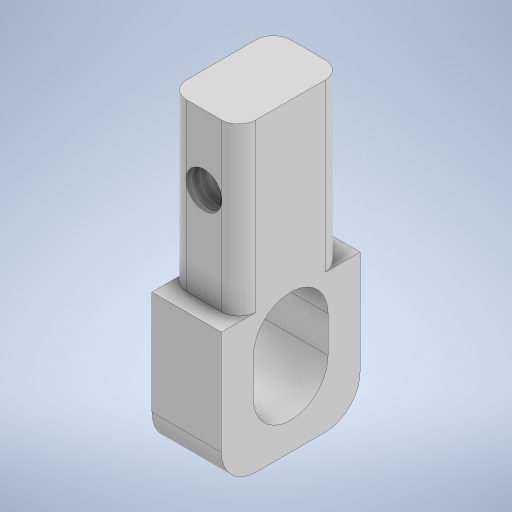
# Autodesk Inventor part: key
Saved by Autodesk Inventor 2023 (Build 270158000, 158)
## iProperties
Created: 2023-01-04
Part Number: key
Material: Generic
Document SubType Name: Modeling
Designer: Hayden Swanson
Density: 1 g/cm^3
Appearance: Default
Author: Hayden Swanson
Autodesk Inventor part; units mm, degrees
ref_plane "YZ Plane" through (0, 0, 0) normal (1, 0, 0) x (0, 1, 0)
ref_plane "XZ Plane" through (0, 0, 0) normal (0, 1, 0) x (-1, 0, 0)
ref_plane "XY Plane" through (0, 0, 0) normal (0, 0, 1) x (1, 0, 0)
sketch "Sketch1" plane through (0, 0, 0) normal (0, 1, 0) x (-1, 0, 0)
  line L0 (0, 0) -> (6.35, 0)
  line L1 (6.35, 0) -> (6.35, -9.525)
  line L2 (6.35, -9.525) -> (0, -9.525)
  line L3 (0, -9.525) -> (0, 0)
  dimension "d0" = 6.35
  dimension "d1" = 9.525
  constraints: 8 end point, 2 parallel, 1 horizontal, 1 perpendicular
  measures "d0" distance of L1.end L2.end
  measures "d1" distance of L0.end L1.end
extrude "Extrusion1" add sketch "Sketch1" along normal blind 27.94
sketch "Sketch3" plane through (-6.35, 0, -9.525) normal (-1, 0, 0) x (0, 0, 1)
  line L0 (0, 0) -> (9.525, 0) projected
  line L1 (0, 0) -> (0, 7.62)
  line L2 (0, 0) -> (0, 27.94) projected
  line L3 (0, 7.62) -> (9.525, 7.62)
  line L4 (4.7625, 2.54) -> (4.7625, 0)
  line L5 (1.5875, 2.54) -> (7.9375, 2.54)
  line L6 (7.9375, 12.7) -> (1.5875, 12.7)
  line L7 (1.5875, 2.54) -> (7.9375, 2.54)
  line L8 (7.9375, 12.7) -> (1.5875, 12.7)
  line L9 (4.7625, 2.54) -> (1.3386, 2.54)
  line L10 (1.3386, 2.54) -> (1.3386, 12.7)
  line L11 (4.7625, 2.54) -> (8.1864, 2.54)
  line L12 (8.1864, 2.54) -> (8.1864, 12.7)
  line L13 (8.1864, 12.7) -> (1.3386, 12.7)
  dimension "d11" = 7.62
  dimension "d32" = 2.54
  dimension "d33" = 10.16
  dimension "d39" = 3.4239
  dimension "d40" = 3.4239
  constraints: 24 end point, 3 horizontal, 2 parallel, 2 perpendicular, 2 point on line, 1 collinear, 1 midpoint
  measures "d11" distance of L0.start L1.end
  measures "d32" distance of L4.start L4.end
  measures "d33" distance of L6.start L5.end
  measures "d39" distance of L4.start L9.end
  measures "d40" distance of L4.start L11.end
extrude "Extrusion3" cut sketch "Sketch3" against normal through all contours L5 L9 L10 L3 L12 L11 | L10 L13 L6 L12 L3
sketch "Sketch4" plane through (0, 0, -9.525) normal (0, 0, -1) x (-1, 0, 0)
  line L0 (0, 0) -> (6.35, 0) projected
  line L1 (0, 0) -> (0, 27.94) projected
  line L2 (6.35, 0) -> (0, 0)
  line L3 (0, 0) -> (0, 12.7)
  line L4 (0, 12.7) -> (6.35, 12.7)
  line L5 (6.35, 12.7) -> (6.35, 0)
  dimension "d22" = 12.7
  constraints: 8 end point, 2 parallel, 1 horizontal, 1 perpendicular, 1 point on line
  measures "d22" distance of L2.end L3.end
extrude "Extrusion4" add sketch "Sketch4" along normal blind 1.5875
sketch "Sketch5" plane through (-6.35, 0, 0) normal (0, 0, 1) x (1, 0, 0)
  line L0 (0, 0) -> (0, 27.94) projected
  line L1 (6.35, 0) -> (0, 0)
  line L2 (0, 0) -> (0, 12.7)
  line L3 (0, 12.7) -> (6.35, 12.7)
  line L4 (6.35, 12.7) -> (6.35, 0)
  dimension "d25" = 12.7
  constraints: 8 end point, 2 parallel, 1 horizontal, 1 perpendicular, 1 point on line
  measures "d25" distance of L1.end L2.end
extrude "Extrusion5" add sketch "Sketch5" along normal blind 1.5875
fillet "Fillet2" radius 3.175 2 edges at (-3.175, 0, 1.5875) (-3.175, 0, -11.1125)
fillet "Fillet5" radius 3.4239 4 edges at (-3.175, 2.54, -8.1864) (-3.175, 2.54, -1.3386) (-3.175, 12.7, -8.1864) (-3.175, 12.7, -1.3386)
fillet "Fillet10" radius 1.5875 4 edges at (-6.35, 20.32, -9.525) (-6.35, 20.32, 0) (0, 20.32, 0) (0, 20.32, -9.525)
sketch "Sketch6" plane through (-4.7625, 27.94, 0) normal (0, 0, 1) x (1, 0, 0)
  line L0 (3.175, 0) -> (0, 0) projected
  line L1 (1.5875, 0) -> (1.5875, -6.35)
  circle A0 centre (1.5875, -6.35) radius 2.0828
  point P0 (4.7625, -27.94)
  dimension "d42" = 6.35
  dimension "d43" = 4.1656
  constraints: 2 end point, 1 centre point, 1 coincident, 1 midpoint, 1 vertical
  measures "d42" distance of L1.start L1.end
  measures "d43" diameter of A0
hole "Hole1" at (-3.175, 21.59, 0) direction (0, 0, -1) diameter 3.302 end through all thread size "8-32 UNC" class "3B" standard "ANSI Unified Screw Threads"
body "Solid1"
